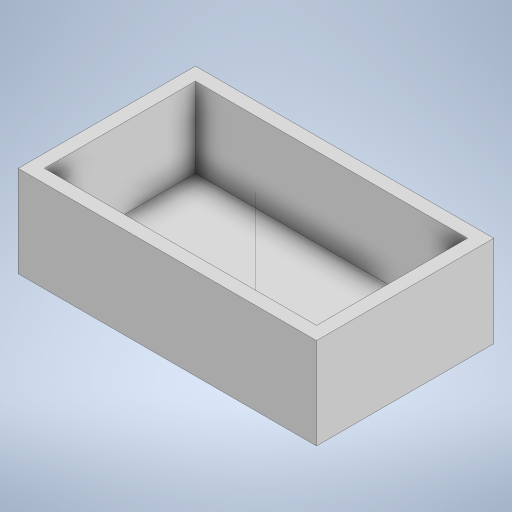
# Autodesk Inventor part: wassertank
Saved by Autodesk Inventor 2023 (Build 270158000, 158)
## iProperties
Created: 2025-06-13
Part Number: wassertank
Material: Generisch
Document SubType Name: Modeling
Designer: johan
Density: 1 g/cm^3
Appearance: Vorgabe
Author: johan
Autodesk Inventor part; units mm, degrees
ref_plane "YZ Plane" through (0, 0, 0) normal (1, 0, 0) x (0, 1, 0)
ref_plane "XZ Plane" through (0, 0, 0) normal (0, 1, 0) x (-1, 0, 0)
ref_plane "XY Plane" through (0, 0, 0) normal (0, 0, 1) x (1, 0, 0)
sketch "Skizze3" plane through (0, 0, 0) normal (0, 0, 1) x (1, 0, 0)
  line L0 (-170, 0) -> (170, 0)
  line L1 (170, 0) -> (170, 104)
  line L2 (170, 104) -> (-170, 104)
  line L3 (-170, 104) -> (-170, 0)
  point P0 (0, 0)
  dimension "d3" = 340
  dimension "d4" = 104
  constraints: 8 end point, 2 parallel, 1 horizontal, 1 perpendicular
  measures "d3" distance of L2.end L1.end
  measures "d4" distance of L1.end L0.end
extrude "Extrusion1" add sketch "Skizze3" along normal mid plane 202
sketch "Skizze4" plane through (-170, 104, 101) normal (0, 1, 0) x (1, 0, 0)
  line L0 (15, 15) -> (325, 15)
  line L1 (325, 15) -> (325, 187)
  line L2 (325, 187) -> (15, 187)
  line L3 (15, 187) -> (15, 15)
  point P0 (170, 101)
  dimension "d7" = 310
  dimension "d8" = 172
  constraints: 8 end point, 2 parallel, 1 horizontal, 1 perpendicular
  measures "d7" distance of L2.end L1.end
  measures "d8" distance of L1.end L0.end
extrude "Extrusion2" cut sketch "Skizze4" against normal blind 91
